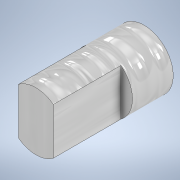
# Autodesk Inventor part: Вал
Saved by Autodesk Inventor 2022 (Build 260153000, 153)
## iProperties
Created: 2022-06-08
Part Number: Вал
Material: Типовые
Document SubType Name: Modeling
Designer: Admin
Density: 1 g/cm^3
Appearance: По умолчанию
Author: Admin
Autodesk Inventor part; units mm, degrees
ref_plane "YZ Plane" through (0, 0, 0) normal (1, 0, 0) x (0, 1, 0)
ref_plane "XZ Plane" through (0, 0, 0) normal (0, 1, 0) x (-1, 0, 0)
ref_plane "XY Plane" through (0, 0, 0) normal (0, 0, 1) x (1, 0, 0)
sketch "Эскиз1" plane through (0, 0, 0) normal (0, 0, 1) x (1, 0, 0)
  circle A0 centre (0, 0) radius 2.5
  line L0 (-1.5, 2) -> (-1.5, -2)
  line L1 (1.5, -2) -> (1.5, 2)
  dimension "d0" = 5
  dimension "d1" = 3
  constraints: 4 end point, 4 point on circle, 2 parallel, 1 centre point, 1 coincident, 1 vertical
  measures "d0" diameter of A0
  measures "d1" distance between parallel lines of L0 L1
extrude "Выдавливание1" add sketch "Эскиз1" along normal blind 7.8 contours L1 A0 L0
extrude "Выдавливание3" add sketch "Эскиз1" against normal blind 1.5
sketch "Эскиз3" plane through (0, 0, 0) normal (0, 0, 1) x (1, 0, 0)
  line L0 (-1.5, 2) -> (-1.5, -2) projected
  arc A0 (-1.5, 2) -> (-1.5, -2) centre (0, 0) ccw projected
  line L1 (1.5, -2) -> (1.5, 2) projected
  arc A1 (1.5, -2) -> (1.5, 2) centre (0, 0) ccw projected
extrude "Выдавливание4" add sketch "Эскиз3" along normal blind 2
